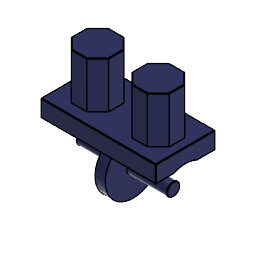
Hips (Autodesk Fusion 360 design; units mm, degrees)
part number: 2026-05-19-13-04-33-670
Autodesk Fusion 360 part; units mm, degrees
sketch "Baseplate" plane through (0, 0, 0) normal (0, 0, 1) x (1, 0, 0)
  line L0 (-7.239, 3.7465) -> (7.239, 3.7465)
  line L1 (7.239, 3.7465) -> (7.239, -3.7465)
  line L2 (7.239, -3.7465) -> (-7.239, -3.7465)
  line L3 (-7.239, -3.7465) -> (-7.239, 3.7465)
  line L4 (-7.239, 3.7465) -> (7.239, -3.7465) construction
  line L5 (7.239, 3.7465) -> (-7.239, -3.7465) construction
  dimension "d1" = 14.478
  dimension "d2" = 7.493
  constraint horizontal L0
  constraint perpendicular L0 L1
  constraint parallel L0 L2
  constraint parallel L1 L3
  constraint coincident L4 origin
  constraint coincident L5 origin
  measures "d1" distance of L1.end L2.end
  measures "d2" distance of L0.end L1.end
extrude "Extrude1" add sketch "Baseplate" against normal blind 2.159
sketch "UpperJoint" plane through (0, 0, 0) normal (0, 0, 1) x (-1, 0, 0)
  line L0 (7.239, 3.7465) -> (-7.239, 3.7465)
  line L1 (-7.239, 3.7465) -> (-7.239, -3.7465)
  line L2 (-7.239, -3.7465) -> (7.239, -3.7465)
  line L3 (7.239, -3.7465) -> (7.239, 3.7465)
  circle A0 centre (-3.81, 0) radius 2.54 construction
  line L4 (-4.782, -2.3467) -> (-2.838, -2.3467)
  line L5 (-2.838, -2.3467) -> (-1.4633, -0.972)
  line L6 (-1.4633, -0.972) -> (-1.4633, 0.972)
  line L7 (-1.4633, 0.972) -> (-2.838, 2.3467)
  line L8 (-2.838, 2.3467) -> (-4.782, 2.3467)
  line L9 (-4.782, 2.3467) -> (-6.1567, 0.972)
  line L10 (-6.1567, 0.972) -> (-6.1567, -0.972)
  line L11 (-6.1567, -0.972) -> (-4.782, -2.3467)
  line L12 (0, -2.5) -> (0, -20)
  line L13 (2.838, 2.3467) -> (4.782, 2.3467)
  line L14 (4.782, 2.3467) -> (6.1567, 0.972)
  line L15 (6.1567, 0.972) -> (6.1567, -0.972)
  line L16 (6.1567, -0.972) -> (4.782, -2.3467)
  line L17 (4.782, -2.3467) -> (2.838, -2.3467)
  line L18 (2.838, -2.3467) -> (1.4633, -0.972)
  line L19 (1.4633, -0.972) -> (1.4633, 0.972)
  line L20 (1.4633, 0.972) -> (2.838, 2.3467)
  point P0 (-3.81, 0)
  dimension "d5" = 5.08
  dimension "d7" = 3.81
  constraint horizontal origin A0.centre
  constraint coincident A0 L4.start
  constraint coincident P0 A0.centre
  constraint horizontal L8
  constraint symmetric L4.start L12 L16.end
  constraint symmetric L4.end L12 L17.end
  constraint symmetric L5.end L12 L18.end
  constraint symmetric L6.end L12 L19.end
  constraint symmetric L7.end L12 L13.start
  constraint symmetric L8.end L12 L13.end
  constraint symmetric L9.end L12 L14.end
  constraint symmetric L10.end L12 L15.end
  measures "d5" diameter of A0
  measures "d7" distance of origin A0.centre
extrude "Extrude2" add sketch "UpperJoint" along normal blind 5.81 contours L4 L5 L6 L7 L8 L9 L10 L11 | L13 L14 L15 L16 L17 L18 L19 L20
sketch "LegJoints" plane through (0, 0, 0) normal (1, 0, 0) x (0, 1, 0)
  circle A0 centre (0, -5.334) radius 3.5052
  dimension "d10" = 7.0104
  dimension "d11" = 5.334
  constraint vertical origin A0.centre
  measures "d10" diameter of A0
  measures "d11" distance of origin A0.centre
extrude "Extrude3" cut sketch "LegJoints" along normal mid plane 20
extrude "Extrude4" add sketch "LegJoints" along normal mid plane 1.3
sketch "LegJoints2" plane through (-0.65, 0, 0) normal (-1, 0, 0) x (0, -1, 0)
  arc A0 (-1.4852, -2.159) -> (1.4852, -2.159) centre (0, -5.334) ccw
  arc A1 (1.4852, -2.159) -> (-1.4852, -2.159) centre (0, -5.334) ccw
  circle A2 centre (0, -5.334) radius 0.8255
  dimension "d16" = 1.651
  constraint coincident A0.centre A1.centre
  measures "d16" diameter of A2
extrude "Extrude5" add sketch "LegJoints2" along normal blind 5.08 contours A2
mirror "Mirror1" about plane through (0, 0, 0) normal (1, 0, 0) of "Extrude5"
fillet "Fillet1" radius 0.0635 2 edges at (5.73, 0.7696, -5.6325) (-5.73, 0.7696, -5.6325) 6 faces at (4.5922, 0.324, 5.81) (-3.0278, -0.324, 5.81) (2.413, 3.7465, -1.4393) (-7.239, 0, -0.6096) (7.239, 0, -0.6096) (-2.413, -3.7465, -1.4393)
named bodies: "Hips"
